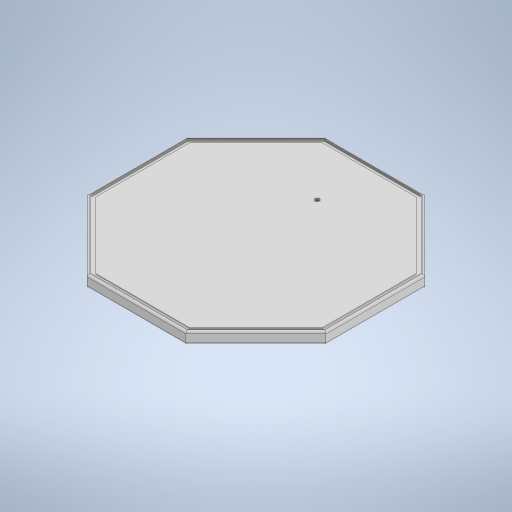
# Autodesk Inventor part: OV-PAM_top_2
Saved by Autodesk Inventor 2024 (Build 280153000, 153)
## iProperties
Created: 2023-06-16
Part Number: OV-PAM_top_2
Material: 일반
Document SubType Name: Modeling
Designer: jsw
Density: 1 g/cm^3
Appearance: 기본값
Author: jsw
Autodesk Inventor part; units mm, degrees
ref_plane "YZ Plane" through (0, 0, 0) normal (1, 0, 0) x (0, 1, 0)
ref_plane "XZ Plane" through (0, 0, 0) normal (0, 1, 0) x (-1, 0, 0)
ref_plane "XY Plane" through (0, 0, 0) normal (0, 0, 1) x (1, 0, 0)
sketch "스케치3" plane through (0, 0, 0) normal (0, 1, 0) x (-1, 0, 0)
  line L0 (68.3838, -28.3255) -> (28.3255, -68.3838)
  line L1 (28.3255, -68.3838) -> (-28.3255, -68.3838)
  line L2 (-28.3255, -68.3838) -> (-68.3838, -28.3255)
  line L3 (-68.3838, -28.3255) -> (-68.3838, 28.3255)
  line L4 (-68.3838, 28.3255) -> (-28.3255, 68.3838)
  line L5 (-28.3255, 68.3838) -> (28.3255, 68.3838)
  line L6 (28.3255, 68.3838) -> (68.3838, 28.3255)
  line L7 (68.3838, 28.3255) -> (68.3838, -28.3255)
  line L8 (65.1838, -27) -> (27, -65.1838)
  line L9 (27, -65.1838) -> (-27, -65.1838)
  line L10 (-27, -65.1838) -> (-65.1838, -27)
  line L11 (-65.1838, -27) -> (-65.1838, 27)
  line L12 (-65.1838, 27) -> (-27, 65.1838)
  line L13 (-27, 65.1838) -> (27, 65.1838)
  line L14 (27, 65.1838) -> (65.1838, 27)
  line L15 (65.1838, 27) -> (65.1838, -27)
  point P0 (0, 0)
  point P1 (0, 0)
  point P2 (0, 0)
  point P3 (0, 0)
  dimension "d43" = 54
  dimension "d44" = 3.2
  constraints: 32 end point, 3 coincident, 2 horizontal, 34 other
  measures "d43" distance of L8.end L9.end
  measures "d44" distance between parallel lines of L7 L15
extrude "돌출2" add sketch "스케치3" along normal blind 6.8 contours L0 L1 L2 L3 L4 L5 L6 L7 | L8 L9 L10 L11 L12 L13 L14 L15
sketch "스케치4" plane through (0, 6.8, 0) normal (0, 1, 0) x (1, 0, 0)
  line L0 (26.9172, -64.9838) -> (-26.9172, -64.9838)
  line L1 (-26.9172, -64.9838) -> (-64.9838, -26.9172)
  line L2 (-64.9838, -26.9172) -> (-64.9838, 26.9172)
  line L3 (-64.9838, 26.9172) -> (-26.9172, 64.9838)
  line L4 (-26.9172, 64.9838) -> (26.9172, 64.9838)
  line L5 (26.9172, 64.9838) -> (64.9838, 26.9172)
  line L6 (64.9838, 26.9172) -> (64.9838, -26.9172)
  line L7 (64.9838, -26.9172) -> (26.9172, -64.9838)
  line L8 (-27.6627, 66.7838) -> (27.6627, 66.7838)
  line L9 (27.6627, 66.7838) -> (66.7838, 27.6627)
  line L10 (66.7838, 27.6627) -> (66.7838, -27.6627)
  line L11 (66.7838, -27.6627) -> (27.6627, -66.7838)
  line L12 (27.6627, -66.7838) -> (-27.6627, -66.7838)
  line L13 (-27.6627, -66.7838) -> (-66.7838, -27.6627)
  line L14 (-66.7838, -27.6627) -> (-66.7838, 27.6627)
  line L15 (-66.7838, 27.6627) -> (-27.6627, 66.7838)
  line L16 (-26.8343, 64.7838) -> (26.8343, 64.7838)
  line L17 (26.8343, 64.7838) -> (64.7838, 26.8343)
  line L18 (64.7838, 26.8343) -> (64.7838, -26.8343)
  line L19 (64.7838, -26.8343) -> (26.8343, -64.7838)
  line L20 (26.8343, -64.7838) -> (-26.8343, -64.7838)
  line L21 (-26.8343, -64.7838) -> (-64.7838, -26.8343)
  line L22 (-64.7838, -26.8343) -> (-64.7838, 26.8343)
  line L23 (-64.7838, 26.8343) -> (-26.8343, 64.7838)
  line L24 (-68.3838, 28.3255) -> (-68.3838, -28.3255) projected
  point P0 (0, 0)
  point P1 (0, 0)
  point P2 (0, 0)
  point P3 (0, 0)
  dimension "d42" = 1.8
  dimension "d45" = 0.2
  dimension "d60" = 1.6
  constraints: 48 end point, 3 coincident, 3 horizontal, 51 other
  measures "d42" distance between parallel lines of L14 L2
  measures "d45" distance between parallel lines of L22 L2
  measures "d60" distance between parallel lines of L24 L14
extrude "돌출3" cut sketch "스케치4" against normal blind 1.2 contours L0 L1 L2 L3 L4 L5 L6 L7 | L8 L9 L10 L11 L12 L13 L14 L15 | L16 L17 L18 L19 L20 L21 L22 L23
sketch "스케치5" plane through (0, 0, 0) normal (0, -1, 0) x (1, 0, 0)
  line L0 (10, 2.5) -> (20, 2.5)
  line L1 (20, 2.5) -> (20, -2.5)
  line L2 (20, -2.5) -> (10, -2.5)
  line L3 (10, -2.5) -> (10, 2.5)
  line L4 (10, 2.5) -> (20, -2.5) construction
  line L5 (20, 2.5) -> (10, -2.5) construction
  line L6 (-20, 2.5) -> (-10, 2.5)
  line L7 (-10, 2.5) -> (-10, -2.5)
  line L8 (-10, -2.5) -> (-20, -2.5)
  line L9 (-20, -2.5) -> (-20, 2.5)
  line L10 (-20, 2.5) -> (-10, -2.5) construction
  line L11 (-10, 2.5) -> (-20, -2.5) construction
  point P0 (0, 0)
  point P1 (15, 0)
  point P2 (-15, 0)
  dimension "d11" = 10
  dimension "d12" = 5
  dimension "d13" = 10
  dimension "d16" = 30
  constraints: 24 end point, 2 horizontal, 2 midpoint, 2 parallel, 1 collinear, 1 horizontal alignment, 1 perpendicular, 10 other
  measures "d11" distance of L1.end L2.end
  measures "d12" distance of L0.end L1.end
  measures "d13" distance from line of L3 point (0, 0)
  measures "d16" distance of L0.start L6.start
extrude "돌출4" add sketch "스케치5" along normal blind 10
sketch "스케치6" plane through (-10, 0, -2.5) normal (0, 0, -1) x (-1, 0, 0)
  circle A0 centre (5, -10) radius 5
  circle A1 centre (-25, -10) radius 5
  line L0 (-20, -10) -> (-30, -10) projected
  line L1 (10, -10) -> (0, -10) projected
  point P0 (-10, 0)
  dimension "d23" = 10
  dimension "d24" = 10
  constraints: 2 centre point, 2 coincident, 2 midpoint
  measures "d23" diameter of A0
  measures "d24" diameter of A1
extrude "돌출5" add sketch "스케치6" against normal blind 5
sketch "스케치7" plane through (-10, 0, -2.5) normal (0, 0, -1) x (-1, 0, 0)
  circle A0 centre (5, -10) radius 1.25
  line L0 (10, 0) -> (10, -10) projected
  line L1 (0, 0) -> (10, 0) projected
  line L2 (4.7788, 0) -> (0, 0)
  circle A1 centre (-25, -10) radius 1.25
  point P0 (-10, 0)
  dimension "d27" = 2.5
  dimension "d28" = 5
  dimension "d31" = 30
  constraints: 2 centre point, 2 end point, 1 horizontal, 1 horizontal alignment, 1 point on line, 2 other
  measures "d27" diameter of A0
  measures "d28" distance from line of L0 A0.centre
  measures "d31" distance of A0.centre A1.centre
extrude "돌출6" cut sketch "스케치7" against normal blind 5
sketch "스케치8" plane through (0, 0, 0) normal (0, -1, 0) x (1, 0, 0)
  circle A0 centre (0, -35) radius 1.25
  line L0 (-10, 2.5) -> (-10, -2.5) projected
  point P0 (0, 0)
  point P1 (-10, 0)
  dimension "d38" = 2.5
  dimension "d39" = 35
  constraints: 1 centre point, 1 midpoint, 1 vertical alignment
  measures "d38" diameter of A0
  measures "d39" vertical distance of A0.centre point (-10, 0)
sketch "스케치9" plane through (0, 5.6, 0) normal (0, 1, 0) x (1, 0, 0)
  line L0 (-26.8343, 64.7838) -> (26.8343, 64.7838)
  line L1 (26.8343, 64.7838) -> (64.7838, 26.8343)
  line L2 (64.7838, 26.8343) -> (64.7838, -26.8343)
  line L3 (64.7838, -26.8343) -> (26.8343, -64.7838)
  line L4 (26.8343, -64.7838) -> (-26.8343, -64.7838)
  line L5 (-26.8343, -64.7838) -> (-64.7838, -26.8343)
  line L6 (-64.7838, -26.8343) -> (-64.7838, 26.8343)
  line L7 (-64.7838, 26.8343) -> (-26.8343, 64.7838)
  line L8 (-27.6627, 66.7838) -> (27.6627, 66.7838) projected
  line L9 (-25.5917, 61.7838) -> (25.5917, 61.7838)
  line L10 (25.5917, 61.7838) -> (61.7838, 25.5917)
  line L11 (61.7838, 25.5917) -> (61.7838, -25.5917)
  line L12 (61.7838, -25.5917) -> (25.5917, -61.7838)
  line L13 (25.5917, -61.7838) -> (-25.5917, -61.7838)
  line L14 (-25.5917, -61.7838) -> (-61.7838, -25.5917)
  line L15 (-61.7838, -25.5917) -> (-61.7838, 25.5917)
  line L16 (-61.7838, 25.5917) -> (-25.5917, 61.7838)
  point P0 (0, 0)
  point P1 (0, 0)
  point P2 (0, 0)
  dimension "d46" = 2
  dimension "d47" = 3
  constraints: 32 end point, 2 coincident, 2 horizontal, 34 other
  measures "d46" distance between parallel lines of L0 L8
  measures "d47" distance between parallel lines of L0 L9
extrude "돌출8" add sketch "스케치9" along normal blind 0.6 contours L0 L1 L2 L3 L4 L5 L6 L7 | L9 L10 L11 L12 L13 L14 L15 L16
fillet "모깎기1" radius 1.2 16 edges at (-68.3838, 6.8, 0) (-48.3546, 6.8, 48.3546) (0, 6.8, 68.3838) (48.3546, 6.8, 48.3546) (68.3838, 6.8, 0) (48.3546, 6.8, -48.3546) (0, 6.8, -68.3838) (-48.3546, 6.8, -48.3546) (48.3546, 0, 48.3546) (0, 0, 68.3838) (-48.3546, 0, 48.3546) (-68.3838, 0, 0) (-48.3546, 0, -48.3546) (0, 0, -68.3838) (48.3546, 0, -48.3546) (68.3838, 0, 0)
sketch "스케치10" plane through (0, 0, 0) normal (0, -1, 0) x (1, 0, 0)
  line L0 (-20, 2.5) -> (-10, 2.5) projected
  line L1 (-10, -2.5) -> (-20, -2.5) projected
  line L2 (-20, 2.5) -> (-19, 2.5)
  line L3 (-19, 2.5) -> (-19, -2.5)
  line L4 (-19, -2.5) -> (-20, -2.5)
  line L5 (-20, -2.5) -> (-20, 2.5)
  line L6 (20, -2.5) -> (10, -2.5) projected
  line L7 (10, 2.5) -> (20, 2.5) projected
  line L8 (20, -2.5) -> (19, -2.5)
  line L9 (19, -2.5) -> (19, 2.5)
  line L10 (19, 2.5) -> (20, 2.5)
  line L11 (20, 2.5) -> (20, -2.5)
  point P0 (0, 0)
  dimension "d54" = 1
  dimension "d55" = 1
  constraints: 16 end point, 4 parallel, 2 horizontal, 2 perpendicular, 2 point on line
  measures "d54" distance of L1.end L3.end
  measures "d55" distance of L9.end L10.end
extrude "돌출9" cut sketch "스케치10" along normal blind 15
extrude "돌출10" cut sketch "스케치8" against normal up to surface (6.2 mm away)
equation "\"d55\" = d54"
